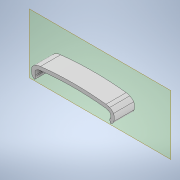
# Autodesk Inventor part: Part3
Saved by Autodesk Inventor 2021 (Build 250183000, 183)
## iProperties
Created: 2021-02-13
Part Number: Part3
Material: Generic
Document SubType Name: Modeling
Designer: user
Density: 1 g/cm^3
Appearance: Default
Author: user
## iProperties of the stored document _3DPrint.ipt
Created: 2021-02-13
Part Number: _3DPrint
Material: Generic
Document SubType Name: Modeling
Designer: user
Density: 1 g/cm^3
Appearance: Default
Author: user
Autodesk Inventor part; units mm, degrees
ref_plane "YZ Plane" through (0, 0, 0) normal (1, 0, 0) x (0, 1, 0)
ref_plane "XZ Plane" through (0, 0, 0) normal (0, 1, 0) x (-1, 0, 0)
ref_plane "XY Plane" through (0, 0, 0) normal (0, 0, 1) x (1, 0, 0)
ref_plane "Work Plane7" through (-1576.3187, -383.5702, 1516.5612) normal (0, 0, 1) x (1, 0, 0)
sketch "Sketch7" plane through (-1576.3187, -383.5702, 1516.5612) normal (0, 0, 1) x (1, 0, 0)
  arc A0 (159.3276, -330.8443) -> (156.2977, -331.6006) centre (159.7307, -338.9062) ccw
  arc A1 (156.2977, -331.6006) -> (153.9729, -333.2489) centre (159.7307, -338.9062) ccw
  arc A2 (153.9729, -333.2489) -> (153.7336, -335.2986) centre (162.867, -335.3261) ccw
  arc A3 (153.7336, -335.2986) -> (153.966, -337.3737) centre (162.867, -335.3261) ccw
  arc A4 (153.966, -337.3737) -> (154.5105, -337.975) centre (154.7761, -337.1873) ccw
  arc A5 (228.4965, -333.0839) -> (226.18, -331.4628) centre (222.6932, -338.9111) ccw
  arc A6 (228.4399, -337.3902) -> (228.4965, -333.0839) centre (220.1875, -335.1281) ccw
  arc A7 (227.7937, -337.975) -> (228.4399, -337.3902) centre (227.6994, -337.2214) ccw
  arc A8 (223.6782, -330.7382) -> (159.3276, -330.8443) centre (191.9649, -610.889) ccw
  arc A9 (226.18, -331.4628) -> (223.6782, -330.7382) centre (222.5826, -339.2015) ccw
  arc A10 (150.5551, -338.1583) -> (153.392, -341.2915) centre (154.7761, -337.1873) ccw
  arc A11 (150.2336, -335.2881) -> (150.5551, -338.1583) centre (162.867, -335.3261) ccw
  arc A12 (150.8193, -331.5239) -> (150.2336, -335.2881) centre (162.867, -335.3261) ccw
  arc A13 (154.8092, -328.4329) -> (150.8193, -331.5239) centre (159.7307, -338.9062) ccw
  arc A14 (159.0274, -327.3556) -> (154.8092, -328.4329) centre (159.7307, -338.9062) ccw
  arc A15 (224.0974, -327.2633) -> (159.0274, -327.3556) centre (191.9649, -610.889) ccw
  arc A16 (227.6596, -328.2909) -> (224.0974, -327.2633) centre (222.5826, -339.2015) ccw
  arc A17 (231.6266, -331.3184) -> (227.6596, -328.2909) centre (222.6932, -338.9111) ccw
  arc A18 (231.8286, -338.2666) -> (231.6266, -331.3184) centre (220.1875, -335.1281) ccw
  arc A19 (228.2282, -341.4479) -> (231.8286, -338.2666) centre (227.6994, -337.2214) ccw
  line L0 (153.392, -341.2915) -> (154.5105, -337.975)
  line L1 (227.7937, -337.975) -> (228.2282, -341.4479)
  point P0 (1576.3187, 383.5702)
  dimension "d20" = 73.2832
  dimension "d21" = 3.5
  dimension "d22" = 74.8362
  constraints: 42 point on circle, 20 centre point, 4 end point, 2 concentric, 2 tangent, 9 other
  measures "d20" distance of L1.start L0.end
  measures "d21" radial gap between concentric circles of A4 A10
  measures "d22" horizontal distance of L1.end L0.start
extrude "Extrusion3" add sketch "Sketch7" along normal blind 20
body "Solid3"
